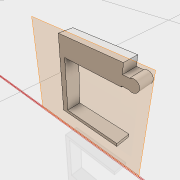
# Autodesk Inventor part: ЛЦМК.00002.00.00.00.00.22 Крышка короба
Saved by Autodesk Inventor 2021.2 (Build 252289000, 289)
## iProperties
Created: 2025-11-20
Part Number: ЛЦМК.00002.00.00.00.00.22 Крышка короба
Material: Типовые
Document SubType Name: Modeling
Designer: Захаров
Density: 1 g/cm^3
Appearance: По умолчанию
Author: Захаров
Autodesk Inventor part; units mm, degrees
ref_plane "YZ Plane" through (0, 0, 0) normal (1, 0, 0) x (0, 1, 0)
ref_plane "XZ Plane" through (0, 0, 0) normal (0, 1, 0) x (-1, 0, 0)
ref_plane "XY Plane" through (0, 0, 0) normal (0, 0, 1) x (1, 0, 0)
ref_plane "РабПлоскость3" through (-23.0229, -31.0507, 3.0679) normal (0, 0, 1) x (1, 0, 0)
sketch "Эскиз2" plane through (-23.0229, -31.0507, 3.0679) normal (0, 0, 1) x (1, 0, 0)
  arc A0 (-1, -3.4852) -> (-1, -0.4852) centre (0, -1.9852) ccw projected
  line L0 (-1, -3.4852) -> (-3, -3.4852) projected
  line L1 (-3, -0.4852) -> (-1, -0.4852) projected
  line L2 (-3, -0.4852) -> (-24.5, -0.4852)
  line L3 (-24.5, -0.4852) -> (-24.5, -3.2999)
  line L4 (-24.5, -3.2999) -> (-1.0821, -3.2999)
  line L5 (-3, -3.2999) -> (-3, -0.4852)
  line L6 (-24.5, -3.2999) -> (-22.5, -3.2999)
  line L7 (-22.5, -3.2999) -> (-22.5, -23.2999)
  line L8 (-22.5, -23.2999) -> (-24.5, -23.2999)
  line L9 (-24.5, -23.2999) -> (-24.5, -3.2999)
  line L10 (-22.5, -23.2999) -> (-3, -23.2999)
  line L11 (-3, -23.2999) -> (-3, -15.9662)
  line L12 (-3, -15.9662) -> (-22.5, -15.9662)
  line L13 (-22.5, -15.9662) -> (-22.5, -23.2999)
  line L14 (-1, -3.2999) -> (-22.5, -3.2999) projected
  line L15 (-22.5, -3.2999) -> (-22.5, -21.2999) projected
  line L16 (-3, -0.5852) -> (-0.9692, -0.5852)
  arc A1 (-1.0821, -3.2999) -> (-0.9692, -0.5852) centre (0, -1.9852) ccw
  line L17 (-0.9692, -3.3852) -> (-1.1358, -3.3852)
  line L18 (-1, -3.2999) -> (-22.5, -3.2999) projected
  line L19 (-22.5, -21.2999) -> (-1, -21.2999) projected
  point P0 (23.0229, 31.0507)
  point P1 (-22.5, -12.2999)
  point P2 (-3, -21.2999)
  point P3 (-22.5, -3.2999)
  point P4 (-3, -0.5852)
  dimension "d3" = 2
  dimension "d4" = 0.1
  dimension "d5" = 2
  constraints: 28 end point, 6 parallel, 5 point on line, 4 point on circle, 3 horizontal, 3 perpendicular, 1 centre point, 1 midpoint
  measures "d3" distance of L7.end L8.end
  measures "d4" radial gap between concentric circles of A0 A1
  measures "d5" distance between parallel lines of L10 L19
extrude "Выдавливание2" add sketch "Эскиз2" against normal blind 15 contours L5 L4 L3 L2 | L16 A1 L4 L5 | L4 L7 L8 L9 | L7 L19 L11 L10
